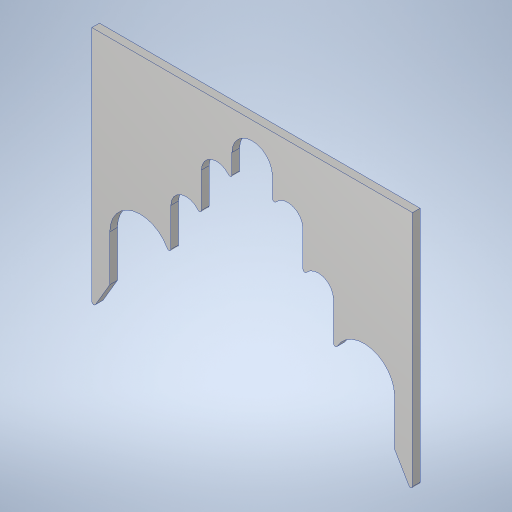
# Autodesk Inventor part: CL1-001
Saved by Autodesk Inventor 2023.4 (Build 274418000, 418)
## iProperties
Created: 2025-01-14
Part Number: CL1-001
Material: Aluminum 6061
Document SubType Name: Modeling
Designer: mavericks
Density: 2.7 g/cm^3
Appearance: Aluminum - Flat
Author: mavericks
Autodesk Inventor part; units mm, degrees
ref_plane "YZ Plane" through (0, 0, 0) normal (1, 0, 0) x (0, 1, 0)
ref_plane "XZ Plane" through (0, 0, 0) normal (0, 1, 0) x (-1, 0, 0)
ref_plane "XY Plane" through (0, 0, 0) normal (0, 0, 1) x (1, 0, 0)
sketch "Sketch1" plane through (0, 0, 0) normal (0, 0, 1) x (1, 0, 0)
  line L0 (-133.35, -101.6) -> (133.35, -101.6) construction
  line L1 (133.35, -101.6) -> (133.35, 101.6) construction
  line L2 (133.35, 101.6) -> (-133.35, 101.6) construction
  line L3 (-133.35, 101.6) -> (-133.35, -101.6) construction
  line L4 (-133.35, -101.6) -> (133.35, 101.6) construction
  line L5 (133.35, -101.6) -> (-133.35, 101.6) construction
  line L6 (-133.35, -101.6) -> (-118.4275, -76.2) construction
  line L7 (-118.4275, -76.2) -> (-118.4275, -38.1) construction
  line L8 (-118.4275, -38.1) -> (-67.6275, -38.1) construction
  line L9 (-67.6275, 6.35) -> (-42.2275, 6.35) construction
  line L10 (-42.2275, 6.35) -> (-42.2275, 44.45) construction
  line L11 (-42.2275, 44.45) -> (-16.8275, 44.45) construction
  line L12 (-16.8275, 44.45) -> (-16.8275, 69.85) construction
  line L13 (-16.8275, 69.85) -> (16.8275, 69.85) construction
  line L14 (16.8275, 69.85) -> (16.8275, 44.45) construction
  line L15 (16.8275, 44.45) -> (42.2275, 44.45) construction
  line L16 (42.2275, 44.45) -> (42.2275, 6.35) construction
  line L17 (42.2275, 6.35) -> (67.6275, 6.35) construction
  line L18 (67.6275, 6.35) -> (67.6275, -38.1) construction
  line L19 (67.6275, -38.1) -> (118.4275, -38.1) construction
  line L20 (118.4275, -38.1) -> (118.4275, -76.2) construction
  line L21 (118.4275, -76.2) -> (133.35, -101.6) construction
  arc A0 (16.8275, 69.85) -> (-16.8275, 69.85) centre (0, 69.85) ccw construction
  arc A1 (-16.8275, 44.45) -> (-42.2275, 44.45) centre (-29.5275, 44.45) ccw construction
  arc A2 (-42.2275, 6.35) -> (-67.6275, 6.35) centre (-54.9275, 6.35) ccw construction
  arc A3 (67.6275, 6.35) -> (42.2275, 6.35) centre (54.9275, 6.35) ccw construction
  arc A4 (42.2275, 44.45) -> (16.8275, 44.45) centre (29.5275, 44.45) ccw construction
  arc A5 (118.4275, -38.1) -> (67.6275, -38.1) centre (93.0275, -38.1) ccw construction
  arc A6 (-67.6275, -38.1) -> (-118.4275, -38.1) centre (-93.0275, -38.1) ccw construction
  line L22 (-67.6275, -38.1) -> (-67.6275, 6.35) construction
  line L23 (-133.35, -101.6) -> (-133.35, 101.6)
  line L24 (133.35, 101.6) -> (-133.35, 101.6)
  line L25 (133.35, 101.6) -> (133.35, -101.6)
  line L26 (133.35, -101.6) -> (118.4275, -76.2)
  line L27 (118.4275, -76.2) -> (118.4275, -38.1)
  arc A7 (118.4275, -38.1) -> (67.6275, -38.1) centre (93.0275, -38.1) ccw
  line L28 (67.6275, -38.1) -> (67.6275, 6.35)
  arc A8 (67.6275, 6.35) -> (42.2275, 6.35) centre (54.9275, 6.35) ccw
  line L29 (42.2275, 6.35) -> (42.2275, 44.45)
  arc A9 (42.2275, 44.45) -> (16.8275, 44.45) centre (29.5275, 44.45) ccw
  line L30 (16.8275, 44.45) -> (16.8275, 69.85)
  arc A10 (16.8275, 69.85) -> (-16.8275, 69.85) centre (0, 69.85) ccw
  line L31 (-16.8275, 69.85) -> (-16.8275, 44.45)
  arc A11 (-16.8275, 44.45) -> (-42.2275, 44.45) centre (-29.5275, 44.45) ccw
  line L32 (-42.2275, 44.45) -> (-42.2275, 6.35)
  arc A12 (-42.2275, 6.35) -> (-67.6275, 6.35) centre (-54.9275, 6.35) ccw
  line L33 (-67.6275, 6.35) -> (-67.6275, -38.1)
  arc A13 (-67.6275, -38.1) -> (-118.4275, -38.1) centre (-93.0275, -38.1) ccw
  line L34 (-118.4275, -38.1) -> (-118.4275, -76.2)
  line L35 (-133.35, -101.6) -> (-118.4275, -76.2)
  point P0 (0, 0)
  dimension "d0" = 266.7
  dimension "d1" = 203.2
  dimension "d3" = 12.7
  dimension "d4" = 12.7
  dimension "d5" = 25.4
  dimension "d7" = 33.655
  dimension "d8" = 90
  dimension "d9" = 90
  dimension "d10" = 90
  dimension "d11" = 25.4
  dimension "d12" = 90
  dimension "d13" = 44.45
  dimension "d14" = 44.45
  dimension "d15" = 25.4
  dimension "d16" = 25.4
  dimension "d17" = 38.1
  dimension "d18" = 38.1
  dimension "d19" = 25.4
  dimension "d21" = 50.8
  dimension "d22" = 50.8
  dimension "d23" = 31.75
  constraints: 72 end point, 28 point on circle, 14 centre point, 9 collinear, 9 midpoint, 9 parallel, 7 coincident, 5 point on line, 3 perpendicular, 1 horizontal, 1 vertical, 1 vertical alignment
  measures "d0" distance of L2.end L1.end
  measures "d1" distance of L1.end L0.end
  measures "d3" radius of A1
  measures "d4" radius of A4
  measures "d5" distance of L10.end L11.end
  measures "d7" distance of L12.end L13.end
  measures "d8" angle of L11 L10
  measures "d9" angle of L9 L22
  measures "d10" angle of L13 L12
  measures "d11" distance of L13.end L14.end
  measures "d12" angle of L13 L14
  measures "d13" distance of L8.end L9.start
  measures "d14" distance of L17.end L18.end
  measures "d15" distance of L9.start L9.end
  measures "d16" distance of L16.end L17.end
  measures "d17" distance of L6.end L7.end
  measures "d18" distance of L19.end L20.end
  measures "d19" vertical distance of L0.start L6.end
  measures "d21" distance of L7.end L8.end
  measures "d22" distance of L18.end L19.end
  measures "d23" distance from line of L2 A0.centre
extrude "Extrusion1" add sketch "Sketch1" along normal blind 6.35
fillet "Fillet1" radius 1.5875 8 edges at (-133.35, -101.6, 3.175) (-67.6275, -38.1, 3.175) (-42.2275, 6.35, 3.175) (-16.8275, 44.45, 3.175) (16.8275, 44.45, 3.175) (42.2275, 6.35, 3.175) (67.6275, -38.1, 3.175) (133.35, -101.6, 3.175)
body "Solid1"
